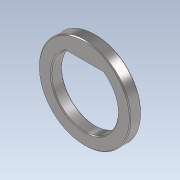
# Autodesk Inventor part: Capston_Distanzscheibe_10mm
Saved by Autodesk Inventor 2022 (Build 260153000, 153)
## iProperties
Created: 2022-07-14
Part Number: Capston_Distanzscheibe_10mm
Material: Edelstahl
Document SubType Name: Modeling
Designer: alexw
Density: 8 g/cm^3
Appearance: Halbpoliert
Mass: 66.7953 g
Surface Area: 44.4232 cm^2
Volume: 8.34941 cm^3
Author: alexw
Autodesk Inventor part; units mm, degrees
ref_plane "YZ Plane" through (0, 0, 0) normal (1, 0, 0) x (0, 1, 0)
ref_plane "XZ Plane" through (0, 0, 0) normal (0, 1, 0) x (-1, 0, 0)
ref_plane "XY Plane" through (0, 0, 0) normal (0, 0, 1) x (1, 0, 0)
sketch "Skizze1" plane through (0, 0, 0) normal (0, 0, 1) x (1, 0, 0)
  circle A0 centre (0, 0) radius 27.5
  circle A1 centre (0, 0) radius 20
  line L0 (-6, 19.0788) -> (-6, 22.8)
  line L1 (-6, 22.8) -> (6, 22.8)
  line L2 (6, 22.8) -> (6, 19.0788)
  line L3 (0, -38.5) -> (0, 38.5) construction
  line L4 (-6, 20) -> (6, 20) construction
  line L5 (-11.3027, 16.5) -> (11.3027, 16.5)
  point P0 (0, 22.8)
  point P1 (0, 20)
  dimension "d0" = 2.8
  dimension "d1" = 12
  dimension "d2" = 40
  dimension "d3" = 55
  dimension "d9" = 3.5
  constraints: 10 end point, 4 point on circle, 3 point on line, 2 centre point, 2 coincident, 2 horizontal, 2 midpoint, 2 perpendicular, 1 tangent, 1 vertical
  measures "d0" distance between parallel lines of L1 L4
  measures "d1" distance between parallel lines of L2 L0
  measures "d2" diameter of A1
  measures "d3" diameter of A0
  measures "d9" distance from line of L5 point (0, 20)
extrude "Extrusion1" add sketch "Skizze1" along normal blind 6.8 contours A0 | L5 A1 | A1 L0 L1 L2 picked at (0.6759, 18.8958)
chamfer "Fase1" distance 0.5 angle 45 6 edges at (-27.5, 0, 6.8) (-27.5, 0, 0) (0, -20, 6.8) (0, 16.5, 6.8) (0, -20, 0) (0, 16.5, 0)
equation "\"d0\" = Nabennuttiefe_20"
equation "\"d1\" = Passfeder_width"
equation "\"d2\" = 2 * Shaft_CapstonPart_Dia"
equation "\"Shaft_CapstonPart_Length\" = 22.8"
equation "\"Nabennuttiefe_20\" = 2.8"
equation "\"Passfeder_width\" = 12"
equation "\"Shaft_CapstonPart_Dia\" = 20"
